Autodesk Fusion 360 part; units mm, degrees
(part 2 of 2)
sketch "top shell" plane through (0, 0, 8) normal (0, 0, 1) x (1, 0, 0) in component "VIC20_diag_up_top"
  line L0 (46.2537, 45.16) -> (52.6038, 45.16) construction
  line L1 (44.825, 45.16) -> (46.2537, 45.16) construction
  line L2 (43.3962, 45.16) -> (44.825, 45.16) construction
  line L3 (43.3962, 24.84) -> (43.3962, 45.16) construction
  line L4 (52.6038, 45.16) -> (52.6038, 37.0638) construction
  line L5 (52.6038, 37.0638) -> (52.6038, 32.9362) construction
  line L6 (52.6038, 32.9362) -> (52.6038, 24.84) construction
  line L7 (52.6038, 24.84) -> (46.2537, 24.84) construction
  line L8 (46.2537, 24.84) -> (44.825, 24.84) construction
  line L9 (44.825, 24.84) -> (43.3962, 24.84) construction
  line L10 (43.3962, 23.62) -> (44.825, 23.62) construction
  line L11 (44.825, 23.62) -> (46.2537, 23.62) construction
  line L12 (46.2537, 23.62) -> (52.6038, 23.62) construction
  line L13 (52.6038, 23.62) -> (52.6038, 17.27) construction
  line L14 (43.3962, 8.38) -> (43.3962, 23.62) construction
  line L15 (44.825, 8.38) -> (43.3962, 8.38) construction
  line L16 (46.2537, 8.38) -> (44.825, 8.38) construction
  line L17 (52.6038, 8.38) -> (46.2537, 8.38) construction
  line L18 (52.6038, 14.73) -> (52.6038, 8.38) construction
  line L19 (52.6038, 17.27) -> (52.6038, 14.73) construction
  circle A0 centre (49, 51) radius 1.5875 construction
  circle A1 centre (57.25, 6.25) radius 1.75 construction
  circle A2 centre (-4.25, 6.25) radius 1.75 construction
  circle A3 centre (4, 51) radius 1.5875 construction
  line L20 (0, 1) -> (0, 54) construction
  line L21 (53, 1) -> (53, 54) construction
  line L22 (60.5, 2) -> (-7.5, 2)
  line L23 (60.5, 0) -> (-7.5, 0)
  arc A4 (-10.5, 3) -> (-7.5, 0) centre (-7.5, 3) ccw
  arc A5 (-8.5, 3) -> (-7.5, 2) centre (-7.5, 3) ccw
  line L24 (-8.5, 3) -> (-8.5, 54.5)
  line L25 (-10.5, 3) -> (-10.5, 54.5)
  arc A6 (-7.5, 55.5) -> (-8.5, 54.5) centre (-7.5, 54.5) ccw
  arc A7 (-7.5, 57.5) -> (-10.5, 54.5) centre (-7.5, 54.5) ccw
  line L26 (-7.5, 57.5) -> (60.5, 57.5)
  line L27 (-7.5, 55.5) -> (60.5, 55.5)
  arc A8 (63.5, 54.5) -> (60.5, 57.5) centre (60.5, 54.5) ccw
  arc A9 (61.5, 54.5) -> (60.5, 55.5) centre (60.5, 54.5) ccw
  line L28 (63.5, 54.5) -> (63.5, 3)
  line L29 (61.5, 54.5) -> (61.5, 3)
  arc A10 (60.5, 0) -> (63.5, 3) centre (60.5, 3) ccw
  arc A11 (60.5, 2) -> (61.5, 3) centre (60.5, 3) ccw
  line L30 (0, 2) -> (0, 0)
  line L31 (53, 2) -> (53, 0)
  arc A12 (62.7, 54.5) -> (60.5, 56.7) centre (60.5, 54.5) ccw
  line L32 (-7.5, 56.7) -> (60.5, 56.7)
  arc A13 (-7.5, 56.7) -> (-9.7, 54.5) centre (-7.5, 54.5) ccw
  line L33 (-9.7, 3) -> (-9.7, 54.5)
  arc A14 (-9.7, 3) -> (-7.5, 0.8) centre (-7.5, 3) ccw
  arc A15 (60.5, 0.8) -> (62.7, 3) centre (60.5, 3) ccw
  line L34 (62.7, 54.5) -> (62.7, 3)
  line L35 (60.5, 0.8) -> (53, 0.8)
  line L36 (0, 0.8) -> (-7.5, 0.8)
  circle A16 centre (4, 51) radius 1.25
  circle A17 centre (57.25, 6.25) radius 1.25
  circle A18 centre (-4.25, 6.25) radius 1.25
  circle A19 centre (49, 51) radius 1.25
  circle A20 centre (4, 51) radius 3.5
  circle A21 centre (49, 51) radius 3.5
  circle A22 centre (57.25, 6.25) radius 3.5
  circle A23 centre (-4.25, 6.25) radius 3.5
  line L37 (43.2962, 7.78) -> (52.7038, 7.78)
  line L38 (53.2038, 8.28) -> (53.2038, 45.26)
  line L39 (52.7038, 45.76) -> (43.2962, 45.76)
  line L40 (42.7962, 45.26) -> (42.7962, 8.28)
  arc A24 (43.2962, 45.76) -> (42.7962, 45.26) centre (43.2962, 45.26) ccw
  arc A25 (53.2038, 45.26) -> (52.7038, 45.76) centre (52.7038, 45.26) ccw
  arc A26 (52.7038, 7.78) -> (53.2038, 8.28) centre (52.7038, 8.28) ccw
  arc A27 (42.7962, 8.28) -> (43.2962, 7.78) centre (43.2962, 8.28) ccw
  line L41 (6.254, 15.746) -> (6.254, 16.254) construction
  line L42 (6.254, 16.254) -> (5.746, 16.254) construction
  line L43 (5.746, 16.254) -> (5.746, 15.746) construction
  line L44 (5.746, 15.746) -> (6.254, 15.746) construction
  line L45 (34.62, 53.175) -> (19.38, 53.175) construction
  line L46 (19.38, 46.825) -> (19.38, 53.175) construction
  line L47 (34.62, 46.825) -> (19.38, 46.825) construction
  line L48 (34.62, 46.825) -> (34.62, 53.175) construction
  line L49 (6.254, 16.254) -> (5.746, 15.746) construction
  line L50 (7.25, 17.75) -> (4.75, 17.75)
  line L51 (4.25, 17.25) -> (4.25, 14.75)
  line L52 (4.75, 14.25) -> (7.25, 14.25)
  line L53 (7.75, 14.75) -> (7.75, 17.25)
  line L54 (7.75, 17.75) -> (4.25, 14.25) construction
  line L55 (4.25, 17.75) -> (7.75, 14.25) construction
  line L56 (19.08, 53.975) -> (34.92, 53.975)
  line L57 (35.42, 53.475) -> (35.42, 46.025)
  line L58 (34.92, 45.525) -> (19.08, 45.525)
  line L59 (18.58, 46.025) -> (18.58, 53.475)
  arc A28 (19.08, 53.975) -> (18.58, 53.475) centre (19.08, 53.475) ccw
  arc A29 (35.42, 53.475) -> (34.92, 53.975) centre (34.92, 53.475) ccw
  arc A30 (34.92, 45.525) -> (35.42, 46.025) centre (34.92, 46.025) ccw
  arc A31 (18.58, 46.025) -> (19.08, 45.525) centre (19.08, 46.025) ccw
  arc A32 (7.75, 17.25) -> (7.25, 17.75) centre (7.25, 17.25) ccw
  arc A33 (7.25, 14.25) -> (7.75, 14.75) centre (7.25, 14.75) ccw
  arc A34 (4.25, 14.75) -> (4.75, 14.25) centre (4.75, 14.75) ccw
  arc A35 (4.75, 17.75) -> (4.25, 17.25) centre (4.75, 17.25) ccw
  point P0 (6, 16)
  dimension "d100" = 0.8
  dimension "d101" = 2.5
  dimension "d102" = 2.5
  dimension "d103" = 2.5
  dimension "d104" = 2.5
  dimension "d105" = 7
  dimension "d106" = 7
  dimension "d107" = 7
  dimension "d108" = 7
  dimension "d113" = 0.6
  dimension "d114" = 0.6
  dimension "d115" = 0.6
  dimension "d116" = 0.6
  dimension "d123" = 0.5
  dimension "d168" = 0.8
  dimension "d169" = 0.8
  dimension "d170" = 0.8
  dimension "d171" = 1.3
  dimension "d172" = 0.5
  dimension "d173" = 0.5
  dimension "d174" = 3.5
  dimension "d175" = 3.5
  constraint coincident L22 L30.start
  constraint coincident L20 L30.start
  constraint coincident L30.end origin
  constraint coincident L22 L31.start
  constraint coincident L21 L31.start
  constraint coincident L23 L31.end
  constraint perpendicular L23 L31
  constraint concentric A8 A12
  constraint concentric A7 A13
  constraint parallel L25 L33
  constraint concentric A4 A14
  constraint parallel L23 L35
  constraint concentric A10 A15
  constraint parallel L28 L34
  constraint tangent A15 L34
  constraint tangent L33 A14
  constraint tangent A12 L34
  constraint tangent A12 L32
  constraint tangent L32 A13
  constraint tangent A13 L33
  constraint tangent A15 L35
  constraint tangent A14 L35
  constraint coincident L31 L35.end
  constraint coincident L30 L36.start
  constraint collinear L35 L36
  constraint concentric A3 A16
  constraint concentric A1 A17
  constraint concentric A2 A18
  constraint concentric A0 A19
  constraint concentric A16 A20
  constraint concentric A19 A21
  constraint concentric A17 A22
  constraint concentric A18 A23
  constraint horizontal L37
  constraint vertical L38
  constraint horizontal L39
  constraint vertical L40
  constraint tangent L39 A24
  constraint tangent L40 A24
  constraint tangent L38 A25
  constraint tangent L39 A25
  constraint equal A24 A25
  constraint tangent L37 A26
  constraint tangent L38 A26
  constraint equal A24 A26
  constraint tangent L37 A27
  constraint tangent L40 A27
  constraint equal A24 A27
  constraint coincident L41.end L42.start
  constraint coincident L43.end L44.start
  constraint horizontal L50
  constraint perpendicular L50 L51
  constraint parallel L50 L52
  constraint parallel L51 L53
  constraint coincident L54 P0
  constraint coincident L55 P0
  constraint midpoint L49 P0
  constraint horizontal L56
  constraint vertical L57
  constraint horizontal L58
  constraint vertical L59
  constraint tangent L56 A28
  constraint tangent L59 A28
  constraint tangent L56 A29
  constraint tangent L57 A29
  constraint equal A28 A29
  constraint tangent L57 A30
  constraint tangent L58 A30
  constraint equal A28 A30
  constraint tangent L58 A31
  constraint tangent L59 A31
  constraint equal A28 A31
  constraint coincident L54.start L50
  constraint coincident L54.start L53
  constraint tangent L50 A32
  constraint tangent L53 A32
  constraint coincident L55.end L53
  constraint coincident L55.end L52
  constraint tangent L53 A33
  constraint tangent L52 A33
  constraint equal A32 A33
  constraint coincident L54.end L52
  constraint coincident L54.end L51
  constraint tangent L52 A34
  constraint tangent L51 A34
  constraint equal A32 A34
  constraint coincident L55.start L51
  constraint coincident L55.start L50
  constraint tangent L51 A35
  constraint tangent L50 A35
  constraint equal A32 A35
  measures "d100" distance of L26 L32
  measures "d101" diameter of A16
  measures "d102" diameter of A17
  measures "d103" diameter of A18
  measures "d104" diameter of A19
  measures "d105" diameter of A20
  measures "d106" diameter of A21
  measures "d107" diameter of A22
  measures "d108" diameter of A23
  measures "d113" distance of L2 L39
  measures "d114" distance of L3 L40
  measures "d115" distance of L4 L38
  measures "d116" distance of L17 L37
  measures "d123" radius of A24
  measures "d168" distance of L45 L56
  measures "d169" distance of L46 L59
  measures "d170" distance of L48 L57
  measures "d171" distance of L47 L58
  measures "d172" radius of A28
  measures "d173" radius of A32
  measures "d174" distance of L50 L52
  measures "d175" distance of L51 L53
extrude "Extrude1''" add sketch "top shell" along normal blind 2 separate body contours L22 A5 L24 A6 L27 A9 L29 A11 L30 L31 A12 L32 A13 L33 A14 A15 L34 L35 L36 | L22 A5 L24 A6 L27 A9 L29 A11 | L22 L23 L30 L31 | L23 A4 L25 A7 L26 A8 L28 A10 L30 L31 A12 L32 A13 L33 A14 A15 L34 L35 L36 | A16 | A17 | A18 | A19 | A20 | A21 | A22 | A23 makes body 11 in component "VIC20_diag_up_top"
extrude "Extrude2''" add sketch "top shell" against normal blind 7.8 contours A20 | A21 bodies 11 in component "VIC20_diag_up_top"
extrude "Extrude3''" add sketch "top shell" against normal blind 7.8 contours A22 | A23 bodies 11 in component "VIC20_diag_up_top"
extrude "Extrude4''" add sketch "top shell" against normal blind 2.5 contours L22 A5 L24 A6 L27 A9 L29 A11 L30 L31 A12 L32 A13 L33 A14 A15 L34 L35 L36 bodies 11 in component "VIC20_diag_up_top"
extrude "Extrude5''" add sketch "top shell" against normal blind 3.5 contours L23 A4 L25 A7 L26 A8 L28 A10 L30 L31 A12 L32 A13 L33 A14 A15 L34 L35 L36 bodies 11 in component "VIC20_diag_up_top"
extrude "Extrude6''" add sketch "top shell" against normal blind 5 contours L22 L23 L30 L31 bodies 11 in component "VIC20_diag_up_top"
fillet "Fillet1'" radius 1 8 edges at (63.5, 28.75, 10) (62.6213, 56.6213, 10) (26.5, 57.5, 10) (-9.6213, 56.6213, 10) (-10.5, 28.75, 10) (-9.6213, 0.8787, 10) (26.5, 0, 10) (62.6213, 0.8787, 10) on bodies 11 in component "VIC20_diag_up_top"
fillet "Fillet4'" radius 0.5 4 edges at (-7.5131, 4.9843, 8) (0.7369, 49.7343, 8) (45.7369, 49.7343, 8) (53.9869, 4.9843, 8) on bodies 11 in component "VIC20_diag_up_top"
fillet "Fillet5'" radius 0.5 8 edges at (-8.5, 28.75, 8) (-8.2071, 55.2071, 8) (26.5, 55.5, 8) (61.2071, 55.2071, 8) (61.5, 28.75, 8) (61.2071, 2.2929, 8) (26.5, 2, 8) (-8.2071, 2.2929, 8) on bodies 11 in component "VIC20_diag_up_top"
chamfer "Chamfer2" distance 0.5 angle 45 14 edges at (51.3338, 12.19, 8.8) (48.7937, 9.65, 8.8) (48.7938, 43.89, 8.8) (51.3338, 40.4769, 8.8) (48.7938, 22.35, 8.8) (51.3338, 19.81, 8.8) (44.6662, 35, 8.8) (44.7456, 43.89, 8.8) (44.7456, 26.11, 8.8) (51.3338, 29.5231, 8.8) (48.7937, 26.11, 8.8) (44.6662, 16, 8.8) (44.7456, 22.35, 8.8) (44.7456, 9.65, 8.8) on bodies 4 5 6 7 8 9 in component "PCB"
extrude "Extrude7" add sketch "DXF VC20_UP" along normal blind 3.5 contours L92 L93 L94 L95 L98 L99 L100 L102 L108 bodies 3 in component "PCB"
extrude "Extrude8" add sketch "DXF VC20_UP" along normal blind 11.2 contours L93 L94 L100 L113 | L95 L99 L102 L113 bodies 3 in component "PCB"
chamfer "Chamfer3" distance 0.75 angle 45 1 edges at (27, 48.095, 11.2) on bodies 3 in component "PCB"
extrude "Extrude9" add sketch "DXF VC20_UP" along normal blind 11 contours L150 L157 L158 L177 | L151 L164 L174 L180 | L152 L153 L156 L160 | L154 L155 L159 L161 | L162 L163 L165 L166 | L170 L171 L175 L176 bodies 3 in component "PCB"
extrude "Extrude10" add sketch "DXF VC20_UP" along normal blind 2.3 contours L61 L69 L71 L77 L81 L89 L90 L91 bodies 3 in component "PCB"
extrude "Extrude11" add sketch "DXF VC20_UP" along normal blind 8.6 contours L189 L196 L203 L232 bodies 3 in component "PCB"
component "PCB" placed x (1, 0, 0) y (0, 1, 0) z (0, 0, 1) at (0, 0, 0)
component "VIC20_diag_up_bottom" placed x (1, 0, 0) y (0, 1, 0) z (0, 0, 1) at (0, 0, 0)
component "VIC20_diag_up_top" placed x (1, 0, 0) y (0, 1, 0) z (0, 0, 1) at (0, 0, 0)
equation "pcb_thickness = 1.6 mm"
equation "below = 2.8 mm + pcb_thickness"
equation "wall = 2 mm"
equation "width = 70 mm + 2 * wall"
equation "length = pcb_length + 0.5 mm + wall"
equation "above = 10 mm - wall"
equation "pcb_width = 53 mm"
equation "pcb_length = 55 mm"
equation "r_corner = 3 mm"
equation "drill = 3.5 mm"
equation "d_screw = 7 mm"
equation "tol_x = 0.3 mm"
equation "tol_connector = 0.6 mm"
equation "d_post = 8.5 mm"
equation "d_post2 = 8 mm"
equation "bottom_height = 4.3 mm + below"
equation "overlap = 1 mm"
equation "top_height = above + below - bottom_height - tol_y"
equation "d34 = -below"
equation "d35 = tol_connector"
equation "d37 = d35"
equation "d47 = length"
equation "d48 = r_corner"
equation "d49 = ( width - pcb_width ) / 2"
equation "d50 = width"
equation "d51 = wall"
equation "d53 = drill"
equation "d54 = d_screw"
equation "d56 = drill"
equation "d57 = d_screw"
equation "d58 = d_post"
equation "d59 = ( width - pcb_width - 2 * wall ) / 4"
equation "d60 = d59"
equation "d61 = drill"
equation "d64 = tol_x"
equation "d65 = tol_x"
equation "d66 = drill"
equation "d67 = d59"
equation "d68 = d67"
equation "d71 = d_post"
equation "d72 = wall * 0.6"
equation "d73 = -wall"
equation "d77 = bottom_height + overlap"
equation "d79 = bottom_height"
equation "d81 = below - pcb_thickness"
equation "d83 = below"
equation "d88 = tol_x"
equation "d89 = d86"
equation "d90 = d87"
equation "d91 = tol_x"
equation "d98 = above"
equation "d100 = wall * 0.4"
equation "d105 = d_screw"
equation "d106 = d_screw"
equation "d107 = d_screw"
equation "d108 = d_screw"
equation "d113 = tol_connector"
equation "d114 = tol_connector"
equation "d115 = tol_connector"
equation "d116 = tol_connector"
equation "d124 = wall"
equation "d126 = -above + tol_y"
equation "d128 = -above + tol_y"
equation "d130 = -top_height + overlap"
equation "d132 = -top_height"
equation "d138 = -top_height - 1.5 mm"
equation "tol_y = 0.2 mm"
equation "d169 = d168"
equation "d170 = d168"
equation "d171 = d168 + 0.5 mm"
named bodies: "PCB", "top shell"
